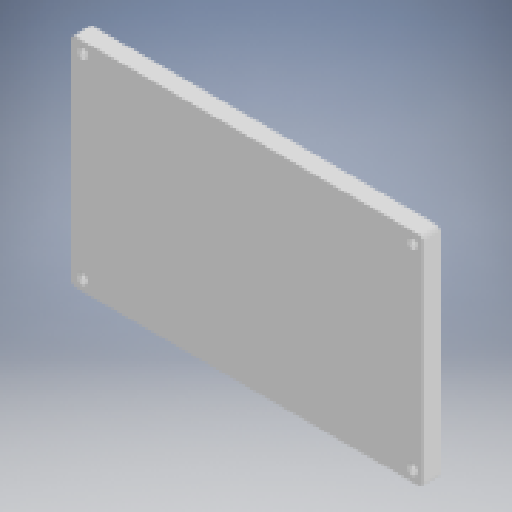
# Autodesk Inventor part: First_Stage_BoxTop_Print
Saved by Autodesk Inventor 2025.2 (Build 292293000, 293)
## iProperties
Created: 2024-12-06
Part Number: First_Stage_BoxTop_Print
Material: Generic
Document SubType Name: Modeling
Designer: Paul Linke
Density: 1 g/cm^3
Appearance: Default
Author: Paul Linke
Autodesk Inventor part; units mm, degrees
ref_plane "YZ Plane" through (0, 0, 0) normal (1, 0, 0) x (0, 1, 0)
ref_plane "XZ Plane" through (0, 0, 0) normal (0, 1, 0) x (-1, 0, 0)
ref_plane "XY Plane" through (0, 0, 0) normal (0, 0, 1) x (1, 0, 0)
sketch "Sketch3" plane through (0, 0, 0) normal (0, 0, 1) x (1, 0, 0)
  line L0 (-8.9702, 53.029) -> (-8.9702, 53.0291) projected
  line L1 (-8.9702, 53.0291) -> (-4.9702, 53.0291) projected
  line L2 (-4.9702, 53.0291) -> (-4.9702, 55.029) projected
  line L3 (-4.9702, 55.029) -> (-87.0018, 55.029) projected
  arc A0 (-87.0018, 55.029) -> (-89.0018, 53.029) centre (-87.0018, 53.029) ccw projected
  line L4 (-89.0018, 53.029) -> (-89.0018, -53.029) projected
  arc A1 (-89.0018, -53.029) -> (-87.0018, -55.029) centre (-87.0018, -53.029) ccw projected
  line L5 (-87.0018, -55.029) -> (-4.9702, -55.029) projected
  line L6 (-4.9702, -55.029) -> (-4.9702, -53.029) projected
  line L7 (-4.9702, -53.029) -> (-8.9702, -53.029) projected
  line L8 (-8.9702, -53.029) -> (-85.0018, -53.029) projected
  arc A2 (-87.0018, -51.029) -> (-85.0018, -53.029) centre (-85.0018, -51.029) ccw projected
  line L9 (-87.0018, -51.029) -> (-87.0018, 51.029) projected
  arc A3 (-85.0018, 53.029) -> (-87.0018, 51.029) centre (-85.0018, 51.029) ccw projected
  line L10 (-85.0018, 53.029) -> (-8.9702, 53.029) projected
  line L11 (49.0298, 53.0291) -> (49.0298, 53.029) projected
  line L12 (49.0298, 53.029) -> (85.0018, 53.029) projected
  arc A4 (87.0018, 51.029) -> (85.0018, 53.029) centre (85.0018, 51.029) ccw projected
  line L13 (87.0018, 51.029) -> (87.0018, -51.029) projected
  arc A5 (85.0018, -53.029) -> (87.0018, -51.029) centre (85.0018, -51.029) ccw projected
  line L14 (85.0018, -53.029) -> (49.0298, -53.029) projected
  line L15 (49.0298, -53.029) -> (45.0298, -53.029) projected
  line L16 (45.0298, -53.029) -> (45.0298, -55.029) projected
  line L17 (45.0298, -55.029) -> (87.0018, -55.029) projected
  arc A6 (87.0018, -55.029) -> (89.0018, -53.029) centre (87.0018, -53.029) ccw projected
  line L18 (89.0018, -53.029) -> (89.0018, 53.029) projected
  arc A7 (89.0018, 53.029) -> (87.0018, 55.029) centre (87.0018, 53.029) ccw projected
  line L19 (87.0018, 55.029) -> (45.0298, 55.029) projected
  line L20 (45.0298, 55.029) -> (45.0298, 53.0291) projected
  line L21 (45.0298, 53.0291) -> (49.0298, 53.0291) projected
  line L22 (87.0018, 55.029) -> (-87.0018, 55.029)
  line L23 (-89.0018, 53.029) -> (-89.0018, -53.029)
  line L24 (-87.0018, -55.029) -> (87.0018, -55.029)
  line L25 (89.0018, -53.029) -> (89.0018, 53.029)
  line L26 (85.1018, 53.129) -> (-85.1018, 53.129)
  line L27 (-87.1018, 51.129) -> (-87.1018, -51.129)
  line L28 (-85.1018, -53.129) -> (85.1018, -53.129)
  line L29 (87.1018, -51.129) -> (87.1018, 51.129)
  arc A8 (89.0018, 53.029) -> (87.0018, 55.029) centre (87.0018, 53.029) ccw
  arc A9 (87.1018, 51.129) -> (85.1018, 53.129) centre (85.1018, 51.129) ccw
  arc A10 (85.1018, -53.129) -> (87.1018, -51.129) centre (85.1018, -51.129) ccw
  arc A11 (87.0018, -55.029) -> (89.0018, -53.029) centre (87.0018, -53.029) ccw
  arc A12 (-87.1018, -51.129) -> (-85.1018, -53.129) centre (-85.1018, -51.129) ccw
  arc A13 (-89.0018, -53.029) -> (-87.0018, -55.029) centre (-87.0018, -53.029) ccw
  arc A14 (-85.1018, 53.129) -> (-87.1018, 51.129) centre (-85.1018, 51.129) ccw
  arc A15 (-87.0018, 55.029) -> (-89.0018, 53.029) centre (-87.0018, 53.029) ccw
  point P0 (0, 0)
  dimension "d0" = 0.1
  dimension "d1" = 0.1
  dimension "d2" = 0.1
  dimension "d3" = 0.1
  dimension "d4" = 2
  constraints: 16 end point, 16 point on circle, 16 tangent, 8 centre point, 7 equal radius, 4 parallel, 2 horizontal, 2 perpendicular
  measures "d0" distance between parallel lines of L9 L27
  measures "d1" distance between parallel lines of L28 L8
  measures "d2" distance between parallel lines of L29 L13
  measures "d3" distance between parallel lines of L26 L12
  measures "d4" radius of A8
extrude "Extrusion1" add sketch "Sketch3" along normal blind 4.2 contours L26 A14 L27 A12 L28 L6 L5 A1 L4 A0 L3 L2 | L2 L22 L20 L26 | L20 L19 A7 L18 A6 L17 L16 L28 A10 L29 A9 L26 | L28 L16 L24 L6
sketch "Sketch4" plane through (0, 0, 4.2) normal (0, 0, 1) x (1, 0, 0)
  line L0 (-87.0018, -55.029) -> (87.0018, -55.029) projected
  arc A0 (87.0018, -55.029) -> (89.0018, -53.029) centre (87.0018, -53.029) ccw projected
  line L1 (89.0018, -53.029) -> (89.0018, 53.029) projected
  arc A1 (89.0018, 53.029) -> (87.0018, 55.029) centre (87.0018, 53.029) ccw projected
  line L2 (87.0018, 55.029) -> (-87.0018, 55.029) projected
  arc A2 (-87.0018, 55.029) -> (-89.0018, 53.029) centre (-87.0018, 53.029) ccw projected
  line L3 (-89.0018, 53.029) -> (-89.0018, -53.029) projected
  arc A3 (-89.0018, -53.029) -> (-87.0018, -55.029) centre (-87.0018, -53.029) ccw projected
  line L4 (85.1018, -53.129) -> (-85.1018, -53.129) projected
  arc A4 (-87.1018, -51.129) -> (-85.1018, -53.129) centre (-85.1018, -51.129) ccw projected
  line L5 (-87.1018, -51.129) -> (-87.1018, 51.129) projected
  arc A5 (-85.1018, 53.129) -> (-87.1018, 51.129) centre (-85.1018, 51.129) ccw projected
  line L6 (-85.1018, 53.129) -> (85.1018, 53.129) projected
  arc A6 (87.1018, 51.129) -> (85.1018, 53.129) centre (85.1018, 51.129) ccw projected
  line L7 (87.1018, 51.129) -> (87.1018, -51.129) projected
  arc A7 (85.1018, -53.129) -> (87.1018, -51.129) centre (85.1018, -51.129) ccw projected
  point P0 (0, 0)
extrude "Extrusion2" add sketch "Sketch4" along normal blind 4.8 contours A3 L3 A2 L2 A1 L1 A0 L0 | L4 A4 L5 A5 L6 A6 L7 A7
sketch "Sketch5" plane through (0, 0, 9) normal (0, 0, 1) x (1, 0, 0)
  circle A0 centre (83.5122, 49.5394) radius 2 projected
  circle A1 centre (83.5122, -49.5394) radius 2 projected
  circle A2 centre (-83.5122, -49.5394) radius 2 projected
  circle A3 centre (-83.5122, 49.5394) radius 2 projected
  circle A4 centre (83.5122, 49.5394) radius 1.45
  circle A5 centre (83.5122, -49.5394) radius 1.45
  circle A6 centre (-83.5122, -49.5394) radius 1.45
  circle A7 centre (-83.5122, 49.5394) radius 1.45
  point P0 (0, 0)
  dimension "d9" = 2.9
  dimension "d10" = 2.9
  dimension "d11" = 2.9
  dimension "d12" = 2.9
  constraints: 4 centre point, 4 coincident
  measures "d9" diameter of A4
  measures "d10" diameter of A5
  measures "d11" diameter of A6
  measures "d12" diameter of A7
extrude "Extrusion3" cut sketch "Sketch5" against normal blind 10 contours A4 | A5 | A6 | A7
chamfer "Chamfer1" distance 1.3 angle 45 4 edges at (82.0622, 49.5394, 9) (82.0622, -49.5394, 9) (-84.9622, 49.5394, 9) (-84.9622, -49.5394, 9)
body "Solid1"
